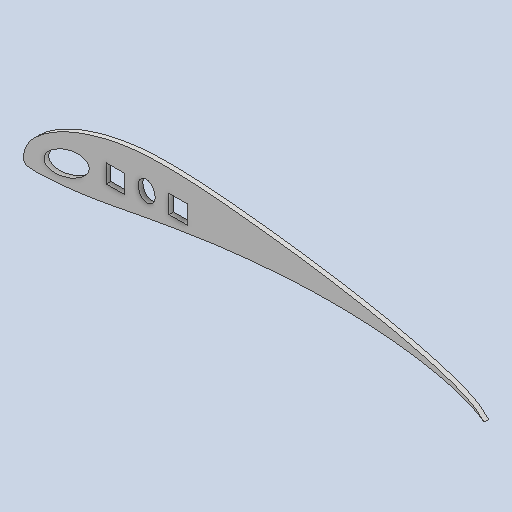
# Autodesk Inventor part: new air foil
Saved by Autodesk Inventor 2024 (Build 280153000, 153)
## iProperties
Created: 2023-07-07
Part Number: new air foil
Material: Generic
Document SubType Name: Modeling
Designer: USER
Density: 1 g/cm^3
Appearance: Default
Author: USER
Autodesk Inventor part; units mm, degrees
ref_plane "YZ Plane" through (0, 0, 0) normal (1, 0, 0) x (0, 1, 0)
ref_plane "XZ Plane" through (0, 0, 0) normal (0, 1, 0) x (-1, 0, 0)
ref_plane "XY Plane" through (0, 0, 0) normal (0, 0, 1) x (1, 0, 0)
sketch "Sketch1" plane through (0, 0, 0) normal (0, 0, 1) x (1, 0, 0)
  spline S0 degree 5 poles (123.1647, -12.7424) (123.1642, -12.7363) (122.9223, -12.5538) (121.8658, -11.7656) (121.7407, -11.4151) (119.4827, -9.5254) (118.2814, -8.4427) (115.4038, -6.7257) (112.5141, -5.4167) (108.5961, -3.7781) (104.3087, -2.2634) (99.2774, -0.6247) (93.7362, 0.9817) (87.6014, 2.6276) (80.9626, 4.255) (73.8309, 5.8737) (66.2625, 7.4614) (58.2945, 9.0198) (49.98, 10.5181) (41.3666, 11.967) (32.5098, 13.3343) (23.46, 14.6343) (14.2858, 15.8497) (5.0441, 16.9757) (-4.1862, 18.031) (-13.3367, 18.9753) (-22.326, 19.8075) (-31.1011, 20.4618) (-39.6031, 20.9306) (-47.8026, 21.1146) (-55.6617, 21.1239) (-63.1272, 20.7542) (-70.2283, 19.9731) (-76.9929, 18.8886) (-83.3929, 17.4592) (-89.4489, 15.7996) (-95.1191, 13.9152) (-100.3884, 11.8726) (-105.2279, 9.6594) (-109.6196, 7.3358) (-113.5447, 4.9251) (-116.9786, 2.4449) (-119.9299, -0.0343) (-122.3434, -2.5383) (-124.1769, -5.0619) (-125.5818, -7.5305) (-126.4379, -9.8471) (-126.9604, -12.0827) (-126.8057, -14.0032) (-126.4732, -15.9508) (-124.4566, -16.5535) (-121.8978, -16.6621) (-118.5563, -16.7771) (-114.5501, -16.5379) (-109.7515, -16.2437) (-104.2431, -15.7036) (-98.0242, -15.012) (-91.177, -14.1289) (-83.7055, -12.8683) (-75.5261, -11.2813) (-66.6565, -9.5956) (-57.1314, -7.802) (-47.0142, -6.0017) (-36.3555, -4.2452) (-25.2576, -2.5964) (-13.7959, -1.1156) (-2.0918, 0.1601) (9.7565, 1.1654) (21.6276, 1.8809) (33.3902, 2.2796) (44.9341, 2.3297) (56.096, 2.0523) (66.8207, 1.4052) (76.8272, 0.5035) (86.3075, -0.8406) (94.5087, -2.1316) (102.5174, -4.187) (108.0429, -5.3476) (114.6006, -8.1812) (116.6902, -8.702) (121.364, -11.6708) (121.3794, -11.5389) (122.8692, -12.5502) (123.1654, -12.7491) (123.1647, -12.7424) knots 0 0 0 0 0 0 0.00602 0.010963 0.017617 0.025421 0.034068 0.043466 0.053614 0.0645 0.07607 0.08826 0.10101 0.114263 0.127966 0.142066 0.156512 0.171254 0.186243 0.201431 0.216768 0.232202 0.247678 0.263136 0.278514 0.293754 0.308799 0.3236 0.338113 0.352315 0.3662 0.379774 0.393048 0.406034 0.418729 0.431115 0.443167 0.454854 0.466145 0.477009 0.48741 0.497336 0.506781 0.515739 0.524204 0.532169 0.539588 0.546561 0.553486 0.560737 0.568651 0.577556 0.587609 0.59865 0.610538 0.623172 0.636501 0.650486 0.665097 0.680307 0.696073 0.712325 0.728985 0.745973 0.76321 0.780614 0.798102 0.81559 0.83299 0.850213 0.867165 0.88375 0.899867 0.915409 0.930259 0.944279 0.957285 0.969034 0.979253 0.98756 0.993452 1 1 1 1 1 1
  line L0 (-47.9037, -0.7293) -> (-37.9037, -0.7293)
  line L1 (-37.9037, -0.7293) -> (-47.9037, -0.7293)
  line L2 (-81.9864, -3.384) -> (-71.9864, -3.384)
  line L3 (-71.9864, -3.384) -> (-81.9864, -3.384)
  line L4 (-81.9864, 6.616) -> (-81.9864, -3.384)
  line L5 (-81.9864, -3.384) -> (-81.9864, 6.616)
  line L6 (-71.9864, -3.384) -> (-81.9864, -3.384)
  line L7 (-81.9864, -3.384) -> (-81.9864, 6.616)
  line L8 (-81.9864, 6.616) -> (-71.9864, 6.616)
  line L9 (-71.9864, 6.616) -> (-71.9864, -3.384)
  line L10 (-81.9864, -3.384) -> (-71.9864, -3.384)
  line L11 (-71.9864, -3.384) -> (-71.9864, 6.616)
  line L12 (-71.9864, 6.616) -> (-81.9864, 6.616)
  line L13 (-81.9864, 6.616) -> (-81.9864, -3.384)
  line L14 (-71.9864, 6.616) -> (-81.9864, 6.616)
  line L15 (-81.9864, 6.616) -> (-71.9864, 6.616)
  line L16 (-37.9037, 9.2707) -> (-37.9037, -0.7293)
  line L17 (-37.9037, -0.7293) -> (-37.9037, 9.2707)
  line L18 (-47.9037, 9.2707) -> (-37.9037, 9.2707)
  line L19 (-37.9037, 9.2707) -> (-47.9037, 9.2707)
  line L20 (-47.9037, -0.7293) -> (-47.9037, 9.2707)
  line L21 (-47.9037, 9.2707) -> (-47.9037, -0.7293)
  ellipse E0 centre (-103.4454, -4.4968) end of major axis (-91.4215, 0.4845) minor radius 6.1868
  line L22 (-37.9037, -0.7293) -> (-37.9037, 9.2707)
  line L23 (-37.9037, 9.2707) -> (-37.9037, -0.7293)
  line L24 (-37.9037, -0.7293) -> (-47.9037, -0.7293)
  line L25 (-47.9037, -0.7293) -> (-47.9037, 9.2707)
  line L26 (-47.9037, 9.2707) -> (-37.9037, 9.2707)
  line L27 (-37.9037, 9.2707) -> (-37.9037, -0.7293)
  line L28 (-47.9037, -0.7293) -> (-37.9037, -0.7293)
  line L29 (-37.9037, -0.7293) -> (-37.9037, 9.2707)
  line L30 (-37.9037, 9.2707) -> (-47.9037, 9.2707)
  line L31 (-47.9037, 9.2707) -> (-47.9037, -0.7293)
  line L32 (-37.9037, 9.2707) -> (-47.9037, 9.2707)
  line L33 (-47.9037, 9.2707) -> (-37.9037, 9.2707)
  line L34 (-47.9037, 9.2707) -> (-47.9037, -0.7293)
  line L35 (-47.9037, -0.7293) -> (-47.9037, 9.2707)
  ellipse E1 centre (-59.9875, 4.2707) end of major axis (-58.8411, -1.1907) minor radius 4.5634
  line L36 (-71.9864, -3.384) -> (-71.9864, 6.616)
  line L37 (-71.9864, 6.616) -> (-71.9864, -3.384)
  line L38 (-81.9864, -3.384) -> (-71.9864, -3.384)
  line L39 (-71.9864, -3.384) -> (-81.9864, -3.384)
  line L40 (-71.9864, -3.384) -> (-71.9864, 6.616)
  line L41 (-71.9864, 6.616) -> (-71.9864, -3.384)
  line L42 (-71.9864, 6.616) -> (-81.9864, 6.616)
  line L43 (-81.9864, 6.616) -> (-71.9864, 6.616)
  line L44 (-81.9864, -3.384) -> (-81.9864, 6.616)
  line L45 (-81.9864, 6.616) -> (-81.9864, -3.384)
  line L46 (-37.9037, -0.7293) -> (-47.9037, -0.7293)
  line L47 (-47.9037, -0.7293) -> (-37.9037, -0.7293)
  point P0 (0, 0)
  point P1 (123.1647, -12.7424)
  point P2 (123.1647, -12.7424)
  constraints: 76 end point, 2 centre point, 31 other
extrude "Extrusion1" add sketch "Sketch1" along normal blind 2.5
body "Solid1"
